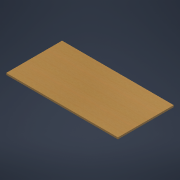
# Autodesk Inventor part: Tabletop
Saved by Autodesk Inventor 2021 (Build 250183000, 183)
## iProperties
Created: 2016-08-30
Part Number: Tabletop
Material: Wood
Document SubType Name: Modeling
Designer: jjsch
Density: 0.570257 g/cm^3
Appearance: Yellow Pine - Solid Natural Low Gloss
Mass: 8000.35 g
Surface Area: 15425.8 cm^2
Volume: 14029.4 cm^3
Author: jjsch
Autodesk Inventor part; units mm, degrees
ref_plane "YZ Plane" through (0, 0, 0) normal (1, 0, 0) x (0, 1, 0)
ref_plane "XZ Plane" through (0, 0, 0) normal (0, 1, 0) x (-1, 0, 0)
ref_plane "XY Plane" through (0, 0, 0) normal (0, 0, 1) x (1, 0, 0)
sketch "Sketch1" plane through (0, 0, 0) normal (0, 1, 0) x (-1, 0, 0)
  line L0 (-609.6, -304.8) -> (609.6, -304.8)
  line L1 (609.6, -304.8) -> (609.6, 304.8)
  line L2 (609.6, 304.8) -> (-609.6, 304.8)
  line L3 (-609.6, 304.8) -> (-609.6, -304.8)
  line L4 (-609.6, -304.8) -> (609.6, 304.8) construction
  line L5 (609.6, -304.8) -> (-609.6, 304.8) construction
  point P0 (0, 0)
  dimension "d0" = 1219.2
  dimension "d1" = 609.6
  constraints: 12 end point, 2 midpoint, 2 parallel, 1 horizontal, 1 perpendicular
  measures "d0" distance of L2.end L1.end
  measures "d1" distance of L1.end L0.end
extrude "Extrusion1" add sketch "Sketch1" along normal blind 19.05
body "Solid1"
